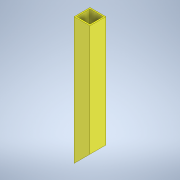
# Autodesk Inventor part: outsideMotorBracket
Saved by Autodesk Inventor 2020.2 (Build 242310000, 310)
## iProperties
Created: 2020-01-18
Part Number: outsideMotorBracket
Material: Aluminum 6061, Welded
Document SubType Name: Modeling
Designer: robst
Density: 2.7 g/cm^3
Appearance: Yellow
Author: robst
Autodesk Inventor part; units mm, degrees
ref_plane "YZ Plane" through (0, 0, 0) normal (1, 0, 0) x (0, 1, 0)
ref_plane "XZ Plane" through (0, 0, 0) normal (0, 1, 0) x (-1, 0, 0)
ref_plane "XY Plane" through (0, 0, 0) normal (0, 0, 1) x (1, 0, 0)
sketch "Sketch1" plane through (0, 0, 0) normal (0, 1, 0) x (-1, 0, 0)
  line L0 (19.05, 19.05) -> (-19.05, 19.05)
  line L1 (-19.05, 19.05) -> (-19.05, -19.05)
  line L2 (-19.05, -19.05) -> (19.05, -19.05)
  line L3 (19.05, -19.05) -> (19.05, 19.05)
  line L4 (19.05, 19.05) -> (-19.05, -19.05) construction
  line L5 (-19.05, 19.05) -> (19.05, -19.05) construction
  line L6 (15.875, 15.875) -> (-15.875, 15.875)
  line L7 (-15.875, 15.875) -> (-15.875, -15.875)
  line L8 (-15.875, -15.875) -> (15.875, -15.875)
  line L9 (15.875, -15.875) -> (15.875, 15.875)
  line L10 (15.875, 15.875) -> (-15.875, -15.875) construction
  line L11 (-15.875, 15.875) -> (15.875, -15.875) construction
  point P0 (0, 0)
  dimension "d0" = 38.1
  dimension "d1" = 38.1
  dimension "d2" = 3.175
  dimension "d3" = 3.175
  constraints: 24 end point, 4 midpoint, 4 parallel, 2 horizontal, 2 perpendicular
  measures "d0" distance of L0.start L0.end
  measures "d1" distance of L1.end L0.end
  measures "d2" distance between parallel lines of L6 L0
  measures "d3" distance between parallel lines of L9 L3
extrude "Extrusion1" add sketch "Sketch1" along normal mid plane 304.8
sketch "Sketch2" plane through (-19.05, 152.4, 19.05) normal (0, 0, 1) x (1, 0, 0)
  line L0 (38.1, -304.8) -> (0, -304.8) projected
  line L1 (0, -304.8) -> (38.1, -266.7)
  line L2 (38.1, -304.8) -> (0, -304.8)
  line L3 (38.1, -304.8) -> (38.1, 0) projected
  line L4 (38.1, -304.8) -> (38.1, -266.7)
  point P0 (19.05, -152.4)
  dimension "d6" = 45
  constraints: 6 end point, 2 point on line
  measures "d6" angle of L1 L0
extrude "Extrusion2" cut sketch "Sketch2" against normal through all
body "Solid1"
